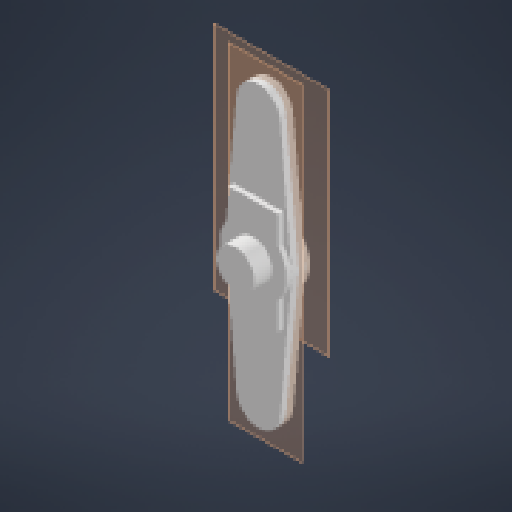
# Autodesk Inventor part: Servo Horn
Saved by Autodesk Inventor 2025.2 (Build 292293000, 293)
## iProperties
Created: 2024-11-18
Part Number: Servo Horn
Material: Generic
Document SubType Name: Modeling
Designer: JL
Density: 1 g/cm^3
Appearance: Default
Author: JL
Autodesk Inventor part; units mm, degrees
ref_plane "YZ Plane" through (0, 0, 0) normal (1, 0, 0) x (0, 1, 0)
ref_plane "XZ Plane" through (0, 0, 0) normal (0, 1, 0) x (-1, 0, 0)
ref_plane "XY Plane" through (0, 0, 0) normal (0, 0, 1) x (1, 0, 0)
ref_plane "Work Plane1" through (223.0039, -4.7048, -1.4) normal (0, 0, 1) x (1, 0, 0)
sketch "Sketch1" plane through (223.0039, -4.7048, -1.4) normal (0, 0, 1) x (1, 0, 0)
  arc A0 (6.5712, 0.3844) -> (6.5712, 1.6156) centre (0, 1) ccw
  line L0 (-6.5712, 0.3844) -> (-4.25, -24.3945)
  arc A1 (-4.25, -24.3945) -> (4.25, -24.3945) centre (0, -23.9964) ccw
  line L1 (4.25, -24.3945) -> (6.5712, 0.3844)
  line L2 (0, 1) -> (-6.6, 1) construction
  line L3 (-6.5712, 1.6156) -> (-4.25, 26.3945)
  arc A2 (4.25, 26.3945) -> (-4.25, 26.3945) centre (0, 25.9964) ccw
  line L4 (4.25, 26.3945) -> (6.5712, 1.6156)
  arc A3 (-6.5712, 0.3844) -> (6.5712, 0.3844) centre (0, 1) ccw construction
  arc A4 (-6.5712, 1.6156) -> (-6.5712, 0.3844) centre (0, 1) ccw
  arc A5 (6.5712, 1.6156) -> (-6.5712, 1.6156) centre (0, 1) ccw construction
  circle A6 centre (0, 1) radius 2.5 construction
  point P0 (-223.0039, 4.7048)
  point P1 (0, -28.265)
  dimension "d0" = 13.2
  dimension "d1" = 8.5
  dimension "d2" = 30
  constraints: 15 point on circle, 10 end point, 7 tangent, 6 centre point, 5 symmetric about line, 1 coincident, 1 horizontal, 1 vertical alignment, 1 other
  measures "d0" diameter of A0
  measures "d1" distance of L1.start L0.end
  measures "d2" distance of L2.end point (0, -28.265)
extrude "Extrusion1" add sketch "Sketch1" along normal blind 2.6
sketch "Sketch2" plane through (223.0039, -4.7048, -1.4) normal (0, 0, -1) x (-1, 0, 0)
  arc A0 (6.5712, 1.6156) -> (-6.5712, 1.6156) centre (0, 1) ccw projected
  arc A1 (-6.5712, 1.6156) -> (-6.5712, 0.3844) centre (0, 1) ccw projected
  arc A2 (-6.5712, 0.3844) -> (6.5712, 0.3844) centre (0, 1) ccw projected
  arc A3 (6.5712, 0.3844) -> (6.5712, 1.6156) centre (0, 1) ccw projected
  line L0 (-4.875, -9) -> (4.875, -9)
  line L1 (4.875, -9) -> (4.875, 11)
  line L2 (4.875, 11) -> (-4.875, 11)
  line L3 (-4.875, 11) -> (-4.875, -9)
  line L4 (-4.875, -9) -> (4.875, 11) construction
  point P0 (4.875, 5.4491)
  point P1 (4.875, -3.4491)
  point P2 (-4.875, -3.4491)
  point P3 (-4.875, 5.4491)
  dimension "d5" = 9.75
  dimension "d6" = 20
  constraints: 10 end point, 2 coincident, 2 parallel, 1 horizontal, 1 midpoint, 1 perpendicular
  measures "d5" distance of L1.end L2.end
  measures "d6" distance of L0.end L1.end
extrude "Extrusion2" add sketch "Sketch2" along normal blind 1
ref_plane "Work Plane2" through (223.0039, -4.7048, -0.1) normal (0, 0, 1) x (1, 0, 0)
mirror "Mirror1" about plane through (223.0039, -4.7048, -0.1) normal (0, 0, 1) of "Extrusion2"
sketch "Sketch3" plane through (218.1289, 6.2952, 2.2) normal (0, 0, 1) x (1, 0, 0)
  arc A0 (0, -5.5509) -> (0, -14.4491) centre (4.875, -10) ccw projected
  arc A1 (0, -5.5509) -> (0, -14.4491) centre (4.875, -10) ccw projected
  circle A2 centre (4.875, -10) radius 3.75
  point P0 (-218.1289, -6.2952)
  point P1 (0, -16.5009)
  point P2 (9.75, -16.5009)
  point P3 (9.75, -14.4491)
  point P4 (9.75, -14.4491)
  point P5 (9.75, 1.9491)
  point P6 (9.75, -5.5509)
  dimension "d9" = 7.5
  constraints: 1 centre point, 1 coincident
  measures "d9" diameter of A2
extrude "Extrusion3" add sketch "Sketch3" along normal blind 3.5
body "Solid1"
